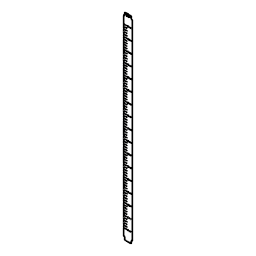
AG10 (Autodesk Fusion 360 design; units mm, degrees)
part number: 2025-10-06-13-20-48-967
Autodesk Fusion 360 part; units mm, degrees
(part 1 of 20)
sketch "Boceto1" plane through (0, 0, 0) normal (0, 1, 0) x (1, 0, 0)
  line L0 (0, 0) -> (40, 0)
  line L1 (40, 0) -> (40, 874)
  line L2 (40, 874) -> (0, 874)
  line L3 (0, 874) -> (0, 0)
  dimension "d1" = 40
  dimension "d2" = 874
  constraint horizontal L0
  constraint vertical L1
  constraint horizontal L2
  constraint vertical L3
  constraint coincident L0.start L3.end
  measures "d1" distance of L1.end L2.end
  measures "d2" distance of L0.end L1.end
extrude "Extruir1" add sketch "Boceto1" along normal blind 3
sketch "Boceto2" plane through (0, 0, 0) normal (0, -1, 0) x (1, 0, 0)
  line L0 (0, 0) -> (0, -874)
  line L1 (0, -874) -> (40, -874)
  line L2 (40, -874) -> (40, 0)
  line L3 (40, 0) -> (0, 0)
  line L4 (0, -836.5) -> (17.5, -836.5)
  line L5 (17.5, -836.5) -> (17.5, -837.5)
  line L6 (17.5, -837.5) -> (0, -837.5)
  line L7 (0, -836.5) -> (0, -837.5)
  line L8 (0, -836.5) -> (0, -837.5)
  line L9 (0, -826.5) -> (17.5, -826.5)
  line L10 (17.5, -827.5) -> (0, -827.5)
  line L11 (0, -826.5) -> (0, -827.5)
  line L12 (17.5, -826.5) -> (17.5, -827.5)
  line L13 (0, -816.5) -> (17.5, -816.5)
  line L14 (17.5, -817.5) -> (0, -817.5)
  line L15 (0, -816.5) -> (0, -817.5)
  line L16 (17.5, -816.5) -> (17.5, -817.5)
  line L17 (0, -806.5) -> (17.5, -806.5)
  line L18 (17.5, -807.5) -> (0, -807.5)
  line L19 (0, -806.5) -> (0, -807.5)
  line L20 (17.5, -806.5) -> (17.5, -807.5)
  line L21 (0, -796.5) -> (17.5, -796.5)
  line L22 (17.5, -797.5) -> (0, -797.5)
  line L23 (0, -796.5) -> (0, -797.5)
  line L24 (17.5, -796.5) -> (17.5, -797.5)
  line L25 (0, -786.5) -> (17.5, -786.5)
  line L26 (17.5, -787.5) -> (0, -787.5)
  line L27 (0, -786.5) -> (0, -787.5)
  line L28 (17.5, -786.5) -> (17.5, -787.5)
  line L29 (0, -776.5) -> (17.5, -776.5)
  line L30 (17.5, -777.5) -> (0, -777.5)
  line L31 (0, -776.5) -> (0, -777.5)
  line L32 (17.5, -776.5) -> (17.5, -777.5)
  line L33 (0, -766.5) -> (17.5, -766.5)
  line L34 (17.5, -767.5) -> (0, -767.5)
  line L35 (0, -766.5) -> (0, -767.5)
  line L36 (17.5, -766.5) -> (17.5, -767.5)
  line L37 (0, -756.5) -> (17.5, -756.5)
  line L38 (17.5, -757.5) -> (0, -757.5)
  line L39 (0, -756.5) -> (0, -757.5)
  line L40 (17.5, -756.5) -> (17.5, -757.5)
  line L41 (0, -746.5) -> (17.5, -746.5)
  line L42 (17.5, -747.5) -> (0, -747.5)
  line L43 (0, -746.5) -> (0, -747.5)
  line L44 (17.5, -746.5) -> (17.5, -747.5)
  line L45 (0, -736.5) -> (17.5, -736.5)
  line L46 (17.5, -737.5) -> (0, -737.5)
  line L47 (0, -736.5) -> (0, -737.5)
  line L48 (17.5, -736.5) -> (17.5, -737.5)
  line L49 (0, -726.5) -> (17.5, -726.5)
  line L50 (17.5, -727.5) -> (0, -727.5)
  line L51 (0, -726.5) -> (0, -727.5)
  line L52 (17.5, -726.5) -> (17.5, -727.5)
  line L53 (0, -716.5) -> (17.5, -716.5)
  line L54 (17.5, -717.5) -> (0, -717.5)
  line L55 (0, -716.5) -> (0, -717.5)
  line L56 (17.5, -716.5) -> (17.5, -717.5)
  line L57 (0, -706.5) -> (17.5, -706.5)
  line L58 (17.5, -707.5) -> (0, -707.5)
  line L59 (0, -706.5) -> (0, -707.5)
  line L60 (17.5, -706.5) -> (17.5, -707.5)
  line L61 (0, -696.5) -> (17.5, -696.5)
  line L62 (17.5, -697.5) -> (0, -697.5)
  line L63 (0, -696.5) -> (0, -697.5)
  line L64 (17.5, -696.5) -> (17.5, -697.5)
  line L65 (0, -686.5) -> (17.5, -686.5)
  line L66 (17.5, -687.5) -> (0, -687.5)
  line L67 (0, -686.5) -> (0, -687.5)
  line L68 (17.5, -686.5) -> (17.5, -687.5)
  line L69 (0, -676.5) -> (17.5, -676.5)
  line L70 (17.5, -677.5) -> (0, -677.5)
  line L71 (0, -676.5) -> (0, -677.5)
  line L72 (17.5, -676.5) -> (17.5, -677.5)
  line L73 (0, -666.5) -> (17.5, -666.5)
  line L74 (17.5, -667.5) -> (0, -667.5)
  line L75 (0, -666.5) -> (0, -667.5)
  line L76 (17.5, -666.5) -> (17.5, -667.5)
  line L77 (0, -656.5) -> (17.5, -656.5)
  line L78 (17.5, -657.5) -> (0, -657.5)
  line L79 (0, -656.5) -> (0, -657.5)
  line L80 (17.5, -656.5) -> (17.5, -657.5)
  line L81 (0, -646.5) -> (17.5, -646.5)
  line L82 (17.5, -647.5) -> (0, -647.5)
  line L83 (0, -646.5) -> (0, -647.5)
  line L84 (17.5, -646.5) -> (17.5, -647.5)
  line L85 (0, -636.5) -> (17.5, -636.5)
  line L86 (17.5, -637.5) -> (0, -637.5)
  line L87 (0, -636.5) -> (0, -637.5)
  line L88 (17.5, -636.5) -> (17.5, -637.5)
  line L89 (0, -626.5) -> (17.5, -626.5)
  line L90 (17.5, -627.5) -> (0, -627.5)
  line L91 (0, -626.5) -> (0, -627.5)
  line L92 (17.5, -626.5) -> (17.5, -627.5)
  line L93 (0, -616.5) -> (17.5, -616.5)
  line L94 (17.5, -617.5) -> (0, -617.5)
  line L95 (0, -616.5) -> (0, -617.5)
  line L96 (17.5, -616.5) -> (17.5, -617.5)
  line L97 (0, -606.5) -> (17.5, -606.5)
  line L98 (17.5, -607.5) -> (0, -607.5)
  line L99 (0, -606.5) -> (0, -607.5)
  line L100 (17.5, -606.5) -> (17.5, -607.5)
  line L101 (0, -596.5) -> (17.5, -596.5)
  line L102 (17.5, -597.5) -> (0, -597.5)
  line L103 (0, -596.5) -> (0, -597.5)
  line L104 (17.5, -596.5) -> (17.5, -597.5)
  line L105 (0, -586.5) -> (17.5, -586.5)
  line L106 (17.5, -587.5) -> (0, -587.5)
  line L107 (0, -586.5) -> (0, -587.5)
  line L108 (17.5, -586.5) -> (17.5, -587.5)
  line L109 (0, -576.5) -> (17.5, -576.5)
  line L110 (17.5, -577.5) -> (0, -577.5)
  line L111 (0, -576.5) -> (0, -577.5)
  line L112 (17.5, -576.5) -> (17.5, -577.5)
  line L113 (0, -566.5) -> (17.5, -566.5)
  line L114 (17.5, -567.5) -> (0, -567.5)
  line L115 (0, -566.5) -> (0, -567.5)
  line L116 (17.5, -566.5) -> (17.5, -567.5)
  line L117 (0, -556.5) -> (17.5, -556.5)
  line L118 (17.5, -557.5) -> (0, -557.5)
  line L119 (0, -556.5) -> (0, -557.5)
  line L120 (17.5, -556.5) -> (17.5, -557.5)
  line L121 (0, -546.5) -> (17.5, -546.5)
  line L122 (17.5, -547.5) -> (0, -547.5)
  line L123 (0, -546.5) -> (0, -547.5)
  line L124 (17.5, -546.5) -> (17.5, -547.5)
  line L125 (0, -536.5) -> (17.5, -536.5)
  line L126 (17.5, -537.5) -> (0, -537.5)
  line L127 (0, -536.5) -> (0, -537.5)
  line L128 (17.5, -536.5) -> (17.5, -537.5)
  line L129 (0, -526.5) -> (17.5, -526.5)
  line L130 (17.5, -527.5) -> (0, -527.5)
  line L131 (0, -526.5) -> (0, -527.5)
  line L132 (17.5, -526.5) -> (17.5, -527.5)
  line L133 (0, -516.5) -> (17.5, -516.5)
  line L134 (17.5, -517.5) -> (0, -517.5)
  line L135 (0, -516.5) -> (0, -517.5)
  line L136 (17.5, -516.5) -> (17.5, -517.5)
  line L137 (0, -506.5) -> (17.5, -506.5)
  line L138 (17.5, -507.5) -> (0, -507.5)
  line L139 (0, -506.5) -> (0, -507.5)
  line L140 (17.5, -506.5) -> (17.5, -507.5)
  line L141 (0, -496.5) -> (17.5, -496.5)
  line L142 (17.5, -497.5) -> (0, -497.5)
  line L143 (0, -496.5) -> (0, -497.5)
  line L144 (17.5, -496.5) -> (17.5, -497.5)
  line L145 (0, -486.5) -> (17.5, -486.5)
  line L146 (17.5, -487.5) -> (0, -487.5)
  line L147 (0, -486.5) -> (0, -487.5)
  line L148 (17.5, -486.5) -> (17.5, -487.5)
  line L149 (0, -476.5) -> (17.5, -476.5)
  line L150 (17.5, -477.5) -> (0, -477.5)
  line L151 (0, -476.5) -> (0, -477.5)
  line L152 (17.5, -476.5) -> (17.5, -477.5)
  line L153 (0, -466.5) -> (17.5, -466.5)
  line L154 (17.5, -467.5) -> (0, -467.5)
  line L155 (0, -466.5) -> (0, -467.5)
  line L156 (17.5, -466.5) -> (17.5, -467.5)
  line L157 (0, -456.5) -> (17.5, -456.5)
  line L158 (17.5, -457.5) -> (0, -457.5)
  line L159 (0, -456.5) -> (0, -457.5)
  line L160 (17.5, -456.5) -> (17.5, -457.5)
  line L161 (0, -446.5) -> (17.5, -446.5)
  line L162 (17.5, -447.5) -> (0, -447.5)
  line L163 (0, -446.5) -> (0, -447.5)
  line L164 (17.5, -446.5) -> (17.5, -447.5)
  line L165 (0, -436.5) -> (17.5, -436.5)
  line L166 (17.5, -437.5) -> (0, -437.5)
  line L167 (0, -436.5) -> (0, -437.5)
  line L168 (17.5, -436.5) -> (17.5, -437.5)
  line L169 (0, -426.5) -> (17.5, -426.5)
  line L170 (17.5, -427.5) -> (0, -427.5)
  line L171 (0, -426.5) -> (0, -427.5)
  line L172 (17.5, -426.5) -> (17.5, -427.5)
  line L173 (0, -416.5) -> (17.5, -416.5)
  line L174 (17.5, -417.5) -> (0, -417.5)
  line L175 (0, -416.5) -> (0, -417.5)
  line L176 (17.5, -416.5) -> (17.5, -417.5)
  line L177 (0, -406.5) -> (17.5, -406.5)
  line L178 (17.5, -407.5) -> (0, -407.5)
  line L179 (0, -406.5) -> (0, -407.5)
  line L180 (17.5, -406.5) -> (17.5, -407.5)
  line L181 (0, -396.5) -> (17.5, -396.5)
  line L182 (17.5, -397.5) -> (0, -397.5)
  line L183 (0, -396.5) -> (0, -397.5)
  line L184 (17.5, -396.5) -> (17.5, -397.5)
  line L185 (0, -386.5) -> (17.5, -386.5)
  line L186 (17.5, -387.5) -> (0, -387.5)
  line L187 (0, -386.5) -> (0, -387.5)
  line L188 (17.5, -386.5) -> (17.5, -387.5)
  line L189 (0, -376.5) -> (17.5, -376.5)
  line L190 (17.5, -377.5) -> (0, -377.5)
  line L191 (0, -376.5) -> (0, -377.5)
  line L192 (17.5, -376.5) -> (17.5, -377.5)
  line L193 (0, -366.5) -> (17.5, -366.5)
  line L194 (17.5, -367.5) -> (0, -367.5)
  line L195 (0, -366.5) -> (0, -367.5)
  line L196 (17.5, -366.5) -> (17.5, -367.5)
  line L197 (0, -356.5) -> (17.5, -356.5)
  line L198 (17.5, -357.5) -> (0, -357.5)
  line L199 (0, -356.5) -> (0, -357.5)
  line L200 (17.5, -356.5) -> (17.5, -357.5)
  line L201 (0, -346.5) -> (17.5, -346.5)
  line L202 (17.5, -347.5) -> (0, -347.5)
  line L203 (0, -346.5) -> (0, -347.5)
  line L204 (17.5, -346.5) -> (17.5, -347.5)
  line L205 (0, -336.5) -> (17.5, -336.5)
  line L206 (17.5, -337.5) -> (0, -337.5)
  line L207 (0, -336.5) -> (0, -337.5)
  line L208 (17.5, -336.5) -> (17.5, -337.5)
  line L209 (0, -326.5) -> (17.5, -326.5)
  line L210 (17.5, -327.5) -> (0, -327.5)
  line L211 (0, -326.5) -> (0, -327.5)
  line L212 (17.5, -326.5) -> (17.5, -327.5)
  line L213 (0, -316.5) -> (17.5, -316.5)
  line L214 (17.5, -317.5) -> (0, -317.5)
  line L215 (0, -316.5) -> (0, -317.5)
  line L216 (17.5, -316.5) -> (17.5, -317.5)
  line L217 (0, -306.5) -> (17.5, -306.5)
  line L218 (17.5, -307.5) -> (0, -307.5)
  line L219 (0, -306.5) -> (0, -307.5)
  line L220 (17.5, -306.5) -> (17.5, -307.5)
  line L221 (0, -296.5) -> (17.5, -296.5)
  line L222 (17.5, -297.5) -> (0, -297.5)
  line L223 (0, -296.5) -> (0, -297.5)
  line L224 (17.5, -296.5) -> (17.5, -297.5)
  line L225 (0, -286.5) -> (17.5, -286.5)
  line L226 (17.5, -287.5) -> (0, -287.5)
  line L227 (0, -286.5) -> (0, -287.5)
  line L228 (17.5, -286.5) -> (17.5, -287.5)
  line L229 (0, -276.5) -> (17.5, -276.5)
  line L230 (17.5, -277.5) -> (0, -277.5)
  line L231 (0, -276.5) -> (0, -277.5)
  line L232 (17.5, -276.5) -> (17.5, -277.5)
  line L233 (0, -266.5) -> (17.5, -266.5)
  line L234 (17.5, -267.5) -> (0, -267.5)
  line L235 (0, -266.5) -> (0, -267.5)
  line L236 (17.5, -266.5) -> (17.5, -267.5)
  line L237 (0, -256.5) -> (17.5, -256.5)
  line L238 (17.5, -257.5) -> (0, -257.5)
  line L239 (0, -256.5) -> (0, -257.5)
  line L240 (17.5, -256.5) -> (17.5, -257.5)
  line L241 (0, -246.5) -> (17.5, -246.5)
  line L242 (17.5, -247.5) -> (0, -247.5)
  line L243 (0, -246.5) -> (0, -247.5)
  line L244 (17.5, -246.5) -> (17.5, -247.5)
  line L245 (0, -236.5) -> (17.5, -236.5)
  line L246 (17.5, -237.5) -> (0, -237.5)
  line L247 (0, -236.5) -> (0, -237.5)
  line L248 (17.5, -236.5) -> (17.5, -237.5)
  line L249 (0, -226.5) -> (17.5, -226.5)
  line L250 (17.5, -227.5) -> (0, -227.5)
  line L251 (0, -226.5) -> (0, -227.5)
  line L252 (17.5, -226.5) -> (17.5, -227.5)
  line L253 (0, -216.5) -> (17.5, -216.5)
  line L254 (17.5, -217.5) -> (0, -217.5)
  line L255 (0, -216.5) -> (0, -217.5)
  line L256 (17.5, -216.5) -> (17.5, -217.5)
  line L257 (0, -206.5) -> (17.5, -206.5)
  line L258 (17.5, -207.5) -> (0, -207.5)
  line L259 (0, -206.5) -> (0, -207.5)
  line L260 (17.5, -206.5) -> (17.5, -207.5)
  line L261 (0, -196.5) -> (17.5, -196.5)
  line L262 (17.5, -197.5) -> (0, -197.5)
  line L263 (0, -196.5) -> (0, -197.5)
  line L264 (17.5, -196.5) -> (17.5, -197.5)
  line L265 (0, -186.5) -> (17.5, -186.5)
  line L266 (17.5, -187.5) -> (0, -187.5)
  line L267 (0, -186.5) -> (0, -187.5)
  line L268 (17.5, -186.5) -> (17.5, -187.5)
  line L269 (0, -176.5) -> (17.5, -176.5)
  line L270 (17.5, -177.5) -> (0, -177.5)
  line L271 (0, -176.5) -> (0, -177.5)
  line L272 (17.5, -176.5) -> (17.5, -177.5)
  line L273 (0, -166.5) -> (17.5, -166.5)
  line L274 (17.5, -167.5) -> (0, -167.5)
  line L275 (0, -166.5) -> (0, -167.5)
  line L276 (17.5, -166.5) -> (17.5, -167.5)
  line L277 (0, -156.5) -> (17.5, -156.5)
  line L278 (17.5, -157.5) -> (0, -157.5)
  line L279 (0, -156.5) -> (0, -157.5)
  line L280 (17.5, -156.5) -> (17.5, -157.5)
  line L281 (0, -146.5) -> (17.5, -146.5)
  line L282 (17.5, -147.5) -> (0, -147.5)
  line L283 (0, -146.5) -> (0, -147.5)
  line L284 (17.5, -146.5) -> (17.5, -147.5)
  line L285 (0, -136.5) -> (17.5, -136.5)
  line L286 (17.5, -137.5) -> (0, -137.5)
  line L287 (0, -136.5) -> (0, -137.5)
  line L288 (17.5, -136.5) -> (17.5, -137.5)
  line L289 (0, -126.5) -> (17.5, -126.5)
  line L290 (17.5, -127.5) -> (0, -127.5)
  line L291 (0, -126.5) -> (0, -127.5)
  line L292 (17.5, -126.5) -> (17.5, -127.5)
  line L293 (0, -116.5) -> (17.5, -116.5)
  line L294 (17.5, -117.5) -> (0, -117.5)
  line L295 (0, -116.5) -> (0, -117.5)
  line L296 (17.5, -116.5) -> (17.5, -117.5)
  line L297 (0, -106.5) -> (17.5, -106.5)
  line L298 (17.5, -107.5) -> (0, -107.5)
  line L299 (0, -106.5) -> (0, -107.5)
  line L300 (17.5, -106.5) -> (17.5, -107.5)
  line L301 (0, -96.5) -> (17.5, -96.5)
  line L302 (17.5, -97.5) -> (0, -97.5)
  line L303 (0, -96.5) -> (0, -97.5)
  line L304 (17.5, -96.5) -> (17.5, -97.5)
  line L305 (0, -86.5) -> (17.5, -86.5)
  line L306 (17.5, -87.5) -> (0, -87.5)
  line L307 (0, -86.5) -> (0, -87.5)
  line L308 (17.5, -86.5) -> (17.5, -87.5)
  line L309 (0, -76.5) -> (17.5, -76.5)
  line L310 (17.5, -77.5) -> (0, -77.5)
  line L311 (0, -76.5) -> (0, -77.5)
  line L312 (17.5, -76.5) -> (17.5, -77.5)
  line L313 (0, -66.5) -> (17.5, -66.5)
  line L314 (17.5, -67.5) -> (0, -67.5)
  line L315 (0, -66.5) -> (0, -67.5)
  line L316 (17.5, -66.5) -> (17.5, -67.5)
  line L317 (0, -56.5) -> (17.5, -56.5)
  line L318 (17.5, -57.5) -> (0, -57.5)
  line L319 (0, -56.5) -> (0, -57.5)
  line L320 (17.5, -56.5) -> (17.5, -57.5)
  line L321 (0, -46.5) -> (17.5, -46.5)
  line L322 (17.5, -47.5) -> (0, -47.5)
  line L323 (0, -46.5) -> (0, -47.5)
  line L324 (17.5, -46.5) -> (17.5, -47.5)
  line L325 (0, -837) -> (35, -837) construction
  line L326 (0, -827) -> (35, -827) construction
  line L327 (0, -817) -> (35, -817) construction
  line L328 (0, -807) -> (35, -807) construction
  line L329 (0, -797) -> (35, -797) construction
  line L330 (0, -787) -> (35, -787) construction
  line L331 (0, -777) -> (35, -777) construction
  line L332 (0, -767) -> (35, -767) construction
  line L333 (0, -757) -> (35, -757) construction
  line L334 (0, -747) -> (35, -747) construction
  line L335 (0, -737) -> (35, -737) construction
  line L336 (0, -727) -> (35, -727) construction
  line L337 (0, -717) -> (35, -717) construction
  line L338 (0, -707) -> (35, -707) construction
  line L339 (0, -697) -> (35, -697) construction
  line L340 (0, -687) -> (35, -687) construction
  line L341 (0, -677) -> (35, -677) construction
  line L342 (0, -667) -> (35, -667) construction
  line L343 (0, -657) -> (35, -657) construction
  line L344 (0, -647) -> (35, -647) construction
  line L345 (0, -637) -> (35, -637) construction
  line L346 (0, -627) -> (35, -627) construction
  line L347 (0, -617) -> (35, -617) construction
  line L348 (0, -607) -> (35, -607) construction
  line L349 (0, -597) -> (35, -597) construction
  line L350 (0, -587) -> (35, -587) construction
  line L351 (0, -577) -> (35, -577) construction
  line L352 (0, -567) -> (35, -567) construction
  line L353 (0, -557) -> (35, -557) construction
  line L354 (0, -547) -> (35, -547) construction
  line L355 (0, -537) -> (35, -537) construction
  line L356 (0, -527) -> (35, -527) construction
  line L357 (0, -517) -> (35, -517) construction
  line L358 (0, -507) -> (35, -507) construction
  line L359 (0, -497) -> (35, -497) construction
  line L360 (0, -487) -> (35, -487) construction
  line L361 (0, -477) -> (35, -477) construction
  line L362 (0, -467) -> (35, -467) construction
  line L363 (0, -457) -> (35, -457) construction
  line L364 (0, -447) -> (35, -447) construction
  line L365 (0, -437) -> (35, -437) construction
  line L366 (0, -427) -> (35, -427) construction
  line L367 (0, -417) -> (35, -417) construction
  line L368 (0, -407) -> (35, -407) construction
  line L369 (0, -397) -> (35, -397) construction
  line L370 (0, -387) -> (35, -387) construction
  line L371 (0, -377) -> (35, -377) construction
  line L372 (0, -367) -> (35, -367) construction
  line L373 (0, -357) -> (35, -357) construction
  line L374 (0, -347) -> (35, -347) construction
  line L375 (0, -337) -> (35, -337) construction
  line L376 (0, -327) -> (35, -327) construction
  line L377 (0, -317) -> (35, -317) construction
  line L378 (0, -307) -> (35, -307) construction
  line L379 (0, -297) -> (35, -297) construction
  line L380 (0, -287) -> (35, -287) construction
  line L381 (0, -277) -> (35, -277) construction
  line L382 (0, -267) -> (35, -267) construction
  line L383 (0, -257) -> (35, -257) construction
  line L384 (0, -247) -> (35, -247) construction
  line L385 (0, -237) -> (35, -237) construction
  line L386 (0, -227) -> (35, -227) construction
  line L387 (0, -217) -> (35, -217) construction
  line L388 (0, -207) -> (35, -207) construction
  line L389 (0, -197) -> (35, -197) construction
  line L390 (0, -187) -> (35, -187) construction
  line L391 (0, -177) -> (35, -177) construction
  line L392 (0, -167) -> (35, -167) construction
  line L393 (0, -157) -> (35, -157) construction
  line L394 (0, -147) -> (35, -147) construction
  line L395 (0, -137) -> (35, -137) construction
  line L396 (0, -127) -> (35, -127) construction
  line L397 (0, -117) -> (35, -117) construction
  line L398 (0, -107) -> (35, -107) construction
  line L399 (0, -97) -> (35, -97) construction
  line L400 (0, -87) -> (35, -87) construction
  line L401 (0, -77) -> (35, -77) construction
  line L402 (0, -67) -> (35, -67) construction
  line L403 (0, -57) -> (35, -57) construction
  line L404 (0, -47) -> (35, -47) construction
  line L405 (0, -36.5) -> (17.5, -36.5)
  line L406 (17.5, -37.5) -> (0, -37.5)
  line L407 (0, -36.5) -> (0, -37.5)
  line L408 (17.5, -36.5) -> (17.5, -37.5)
  line L409 (0, -37) -> (35, -37) construction
  dimension "d11" = 0
  dimension "d12" = 800
  dimension "d34" = 0
  dimension "d35" = 800
  constraint midpoint L8 L325.start
sketch "Boceto5" plane through (0, 0, 0) normal (0, -1, 0) x (1, 0, 0)
  line L0 (17.5002, -789) -> (35.0197, -788.9987) construction
  line L1 (35.0197, -788.9987) -> (35.0194, -784.9987) construction
  line L2 (35.0194, -784.9987) -> (17.4998, -785) construction
  line L3 (17.4998, -785) -> (17.5002, -789) construction
  line L4 (17.5, -739) -> (35.0058, -738.9996) construction
  line L5 (35.0058, -738.9996) -> (35.0057, -734.9996) construction
  line L6 (35.0057, -734.9996) -> (17.5, -735) construction
  line L7 (17.5, -735) -> (17.5, -739) construction
  line L8 (17.5, -689) -> (35.0027, -688.9998) construction
  line L9 (35.0027, -688.9998) -> (35.0027, -684.9998) construction
  line L10 (35.0027, -684.9998) -> (17.5, -685) construction
  line L11 (17.5, -685) -> (17.5, -689) construction
  line L12 (17.5001, -639) -> (35.0059, -638.9995) construction
  line L13 (35.0059, -638.9995) -> (35.0057, -634.9995) construction
  line L14 (35.0057, -634.9995) -> (17.4999, -635) construction
  line L15 (17.4999, -635) -> (17.5001, -639) construction
  line L16 (17.5, -589) -> (35.001, -588.9999) construction
  line L17 (35.001, -588.9999) -> (35.0009, -584.9999) construction
  line L18 (35.0009, -584.9999) -> (17.5, -585) construction
  line L19 (17.5, -585) -> (17.5, -589) construction
  line L20 (17.5002, -539) -> (35.0154, -538.9985) construction
  line L21 (35.0154, -538.9985) -> (35.015, -534.9985) construction
  line L22 (35.015, -534.9985) -> (17.4998, -535) construction
  line L23 (17.4998, -535) -> (17.5002, -539) construction
  line L24 (17.5, -489) -> (35.0025, -488.9997) construction
  line L25 (35.0025, -488.9997) -> (35.0025, -484.9997) construction
  line L26 (35.0025, -484.9997) -> (17.5, -485) construction
  line L27 (17.5, -485) -> (17.5, -489) construction
  line L28 (17.5002, -439) -> (35.0113, -438.9986) construction
  line L29 (35.0113, -438.9986) -> (35.0109, -434.9986) construction
  line L30 (35.0109, -434.9986) -> (17.4998, -435) construction
  line L31 (17.4998, -435) -> (17.5002, -439) construction
  line L32 (17.5, -389) -> (35.002, -388.9997) construction
  line L33 (35.002, -388.9997) -> (35.0019, -384.9997) construction
  line L34 (35.0019, -384.9997) -> (17.5, -385) construction
  line L35 (17.5, -385) -> (17.5, -389) construction
  line L36 (17.5001, -339) -> (35.0028, -338.9996) construction
  line L37 (35.0028, -338.9996) -> (35.0027, -334.9996) construction
  line L38 (35.0027, -334.9996) -> (17.4999, -335) construction
  line L39 (17.4999, -335) -> (17.5001, -339) construction
  line L40 (17.5, -289) -> (35.0002, -289) construction
  line L41 (35.0002, -289) -> (35.0002, -285) construction
  line L42 (35.0002, -285) -> (17.5, -285) construction
  line L43 (17.5, -285) -> (17.5, -289) construction
  line L44 (17.5, -239) -> (34.9994, -239.0001) construction
  line L45 (34.9994, -239.0001) -> (34.9994, -235.0001) construction
  line L46 (34.9994, -235.0001) -> (17.5, -235) construction
  line L47 (17.5, -235) -> (17.5, -239) construction
  line L48 (17.5, -189) -> (35, -189) construction
  line L49 (35, -189) -> (35, -185) construction
  line L50 (35, -185) -> (17.5, -185) construction
  line L51 (17.5, -185) -> (17.5, -189) construction
  line L52 (17.5, -139) -> (35, -139) construction
  line L53 (35, -139) -> (35, -135) construction
  line L54 (35, -135) -> (17.5, -135) construction
  line L55 (17.5, -135) -> (17.5, -139) construction
  line L56 (17.5, -89) -> (35, -89) construction
  line L57 (35, -89) -> (35, -85) construction
  line L58 (35, -85) -> (17.5, -85) construction
  line L59 (17.5, -85) -> (17.5, -89) construction
  line L60 (17.5, -39) -> (35, -39) construction
  line L61 (35, -39) -> (35, -35) construction
  line L62 (35, -35) -> (17.5, -35) construction
  line L63 (17.5, -35) -> (17.5, -39) construction
  line L64 (0, -827) -> (35, -827) construction
  line L65 (17.5001, -839) -> (35.0094, -838.9994) construction
  line L66 (35.0094, -838.9994) -> (35.0093, -834.9994) construction
  line L67 (35.0093, -834.9994) -> (17.4999, -835) construction
  line L68 (17.4999, -835) -> (17.5001, -839) construction
  dimension "d93" = 5
  dimension "d94" = 0
  dimension "d103" = 5
  dimension "d104" = 0
  dimension "d113" = 5
  dimension "d114" = 0
  dimension "d123" = 5
  dimension "d124" = 0
  dimension "d133" = 5
  dimension "d134" = 0
  dimension "d143" = 5
  dimension "d144" = 0
  dimension "d153" = 5
  dimension "d154" = 0
  dimension "d163" = 5
  dimension "d164" = 0
  dimension "d173" = 5
  dimension "d174" = 0
  dimension "d183" = 5
  dimension "d184" = 0
  dimension "d193" = 5
  dimension "d194" = 0
  dimension "d203" = 5
  dimension "d204" = 0
  dimension "d213" = 5
  dimension "d214" = 0
  dimension "d223" = 5
  dimension "d224" = 0
  dimension "d233" = 5
  dimension "d234" = 0
  dimension "d243" = 5
  dimension "d244" = 0
  dimension "d245" = 5
  dimension "d246" = 0
  text T0 "5 cm" font "Arial" height 5 align centre middle in box 17.5196 x 4 at (17.5002, -789) x (1, 0.000075) y (-0.000075, 1) spacing 1 kerned
  text T1 "10cm" font "Arial" height 5 align centre middle in box 17.5057 x 4 at (17.5, -739) x (1, 0.000024) y (-0.000024, 1) spacing 1 kerned
  text T2 "15cm" font "Arial" height 5 align centre middle in box 17.5027 x 4 at (17.5, -689) x (1, 0.000012) y (-0.000012, 1) spacing 1 kerned
  text T3 "20cm" font "Arial" height 5 align centre middle in box 17.5058 x 4 at (17.5001, -639) x (1, 0.000028) y (-0.000028, 1) spacing 1 kerned
  text T4 "25cm" font "Arial" height 5 align centre middle in box 17.501 x 4 at (17.5, -589) x (1, 0.000005) y (-0.000005, 1) spacing 1 kerned
  text T5 "30cm" font "Arial" height 5 align centre middle in box 17.5152 x 4 at (17.5002, -539) x (1, 0.000086) y (-0.000086, 1) spacing 1 kerned
  text T6 "35cm" font "Arial" height 5 align centre middle in box 17.5025 x 4 at (17.5, -489) x (1, 0.000016) y (-0.000016, 1) spacing 1 kerned
  text T7 "40cm" font "Arial" height 5 align centre middle in box 17.5111 x 4 at (17.5002, -439) x (1, 0.000077) y (-0.000077, 1) spacing 1 kerned
  text T8 "45cm" font "Arial" height 5 align centre middle in box 17.5019 x 4 at (17.5, -389) x (1, 0.000015) y (-0.000015, 1) spacing 1 kerned
  text T9 "50cm" font "Arial" height 5 align centre middle in box 17.5028 x 4 at (17.5001, -339) x (1, 0.000025) y (-0.000025, 1) spacing 1 kerned
  text T10 "55cm" font "Arial" height 5 align centre middle in box 17.5002 x 4 at (17.5, -289) x (1, 0.000002) y (-0.000002, 1) spacing 1 kerned
  text T11 "60cm" font "Arial" height 5 align centre middle in box 17.4994 x 4 at (17.5, -239) x (1, -0.000008) y (0.000008, 1) spacing 1 kerned
  text T12 "65cm" font "Arial" height 5 align centre middle in box 17.5 x 4 at (17.5, -189) x (1, 0) y (0, 1) spacing 1 kerned
  text T13 "70cm" font "Arial" height 5 align centre middle in box 17.5 x 4 at (17.5, -139) x (1, -0.000001) y (0.000001, 1) spacing 1 kerned
  text T14 "75cm" font "Arial" height 5 align centre middle in box 17.5 x 4 at (17.5, -89) x (1, 0.000001) y (-0.000001, 1) spacing 1 kerned
  text T15 "80cm" font "Arial" height 5 align centre middle in box 17.5 x 4 at (17.5, -39) x (1, -0.000001) y (0.000001, 1) spacing 1 kerned
  text T16 "0 cm" font "Arial" height 5 align centre middle in box 17.5094 x 4 at (17.5001, -839) x (1, 0.000035) y (-0.000035, 1) spacing 1 kerned
sketch "Boceto6" plane through (0, 0, 0) normal (0, -1, 0) x (1, 0, 0)
  line L0 (0, 0) -> (0, -874)
  line L1 (0, -874) -> (40, -874)
  line L2 (40, -874) -> (40, 0)
  line L3 (40, 0) -> (0, 0)
  line L4 (40, 0) -> (35, 0)
  line L5 (35, 0) -> (35, -3)
  line L6 (35, -3) -> (40, -3)
  line L7 (40, -3) -> (40, 0)
  line L8 (0, 0) -> (5, 0)
  line L9 (5, 0) -> (5, -3)
  line L10 (5, -3) -> (0, -3)
  line L11 (0, -3) -> (0, 0)
  constraint horizontal L4
  constraint vertical L5
  constraint horizontal L6
  constraint vertical L7
  constraint coincident L2.end L3.start
  constraint horizontal L8
  constraint vertical L9
  constraint horizontal L10
  constraint vertical L11
  constraint coincident L0.start L3.end
extrude "Extruir3" cut sketch "Boceto6" against normal blind 3 contours L0 L3 L8 L9 L10 L11 | L2 L3 L4 L5 L6 L7
sketch "Boceto7" plane through (0, 0, 0) normal (0, -1, 0) x (1, 0, 0)
  line L0 (5, -3) -> (0, -3)
  line L1 (0, -3) -> (0, -874)
  line L2 (0, -874) -> (40, -874)
  line L3 (40, -874) -> (40, -3)
  line L4 (40, -3) -> (35, -3)
  line L5 (35, -3) -> (35, 0)
  line L6 (35, 0) -> (5, 0)
  line L7 (5, 0) -> (5, -3)
  line L8 (40, -874) -> (35, -874)
  line L9 (35, -874) -> (35, -870.7)
  line L10 (35, -870.7) -> (40, -870.7)
  line L11 (40, -870.7) -> (40, -874)
  line L12 (0, -874) -> (5, -874)
  line L13 (5, -874) -> (5, -870.7)
  line L14 (5, -870.7) -> (0, -870.7)
  line L15 (0, -870.7) -> (0, -874)
  dimension "d251" = 5
  dimension "d252" = 5
  dimension "d255" = 3.3
  dimension "d256" = 3.3
  constraint horizontal L8
  constraint vertical L9
  constraint horizontal L10
  constraint vertical L11
  constraint coincident L2.end L3.start
  constraint horizontal L12
  constraint vertical L13
  constraint horizontal L14
  constraint vertical L15
  constraint coincident L1.end L2.start
  measures "d251" distance of L13.end L14.end
  measures "d252" distance of L9.end L10.end
  measures "d255" distance of L2.end L10.end
  measures "d256" distance of L1.end L14.end
extrude "Extruir4" cut sketch "Boceto7" along normal mid plane 40 contours L1 L2 L12 L13 L14 L15 | L2 L3 L8 L9 L10 L11
sketch "Boceto8" plane through (0, 0, 0) normal (0, 1, 0) x (1, 0, 0)
extrude "Extruir5" add sketch "Boceto2" along normal blind 1 contours L0 L1 L2 L3 L4 L5 L6 L9 L10 L12 L13 L14 L16 L17 L18 L20 L21 L22 L24 L25 L26 L28 L29 L30 L32 L33 L34 L36 L37 L38 L40 L41 L42 L44 L45 L46 L48 L49 L50 L52 L53 L54 L56 L57 L58 L60 L61 L62 L64 L65 L66 L68 L69 L70 L72 L73 L74 L76 L77 L78 L80 L81 L82 L84 L85 L86 L88 L89 L90 L92 L93 L94 L96 L97 L98 L100 L101 L102 L104 L105 L106 L108 L109 L110 L112 L113 L114 L116 L117 L118 L120 L121 L122 L124 L125 L126 L128 L129 L130 L132 L133 L134 L136 L137 L138 L140 L141 L142 L144 L145 L146 L148 L149 L150 L152 L153 L154 L156 L157 L158 L160 L161 L162 L164 L165 L166 L168 L169 L170 L172 L173 L174 L176 L177 L178 L180 L181 L182 L184 L185 L186 L188 L189 L190 L192 L193 L194 L196 L197 L198 L200 L201 L202 L204 L205 L206 L208 L209 L210 L212 L213 L214 L216 L217 L218 L220 L221 L222 L224 L225 L226 L228 L229 L230 L232 L233 L234 L236 L237 L238 L240 L241 L242 L244 L245 L246 L248 L249 L250 L252 L253 L254 L256 L257 L258 L260 L261 L262 L264 L265 L266 L268 L269 L270 L272 L273 L274 L276 L277 L278 L280 L281 L282 L284 L285 L286 L288 L289 L290 L292 L293 L294 L296 L297 L298 L300 L301 L302 L304 L305 L306 L308 L309 L310 L312 L313 L314 L316 L317 L318 L320 L321 L322 L324 L405 L406 L408
extrude "Extruir6" cut 1 faces at (25, 3, -292.2333) along direction (0, -1, 0) blind 1
extrude "Extruir7" cut sketch "Boceto5" along normal blind 1 text T15 T14 T13 T12 T11 T10 T9 T8 T7 T6 T5 T4 T3 T2 T1 T0 T16
extrude "Extruir8" cut 4 faces at (3.3333, 0, -871.8) (36.6667, 0, -871.8) (1.6667, 0, -1) (36.6667, 0, -1) along direction (0, -1, 0) blind 20
sketch "Boceto10" plane through (0, -1, 0) normal (0, -1, 0) x (1, 0, 0)
  line L0 (28.545, -839.4996) -> (28.5449, -835.8775)
  line L1 (28.5449, -835.8775) -> (29.094, -835.8775)
  line L2 (29.094, -835.8775) -> (29.094, -836.3857)
  spline S0 degree 3 poles (29.094, -836.3857) (29.1559, -836.3011) (29.2808, -836.1306) (29.4582, -836.0156) (29.5476, -835.9576) knots 0 0 0 0 0.031158 0.062835 0.062835 0.062835 0.062835
  spline S1 degree 3 poles (29.5476, -835.9576) (29.6468, -835.9104) (29.8507, -835.8133) (30.0763, -835.8016) (30.1922, -835.7956) knots 0 0 0 0 0.032617 0.067048 0.067048 0.067048 0.067048
  spline S2 degree 3 poles (30.1922, -835.7956) (30.3167, -835.8003) (30.5491, -835.8092) (30.7561, -835.914) (30.8522, -835.9627) knots 0 0 0 0 0.036859 0.068796 0.068796 0.068796 0.068796
  spline S3 degree 3 poles (30.8522, -835.9627) (30.9319, -836.0244) (31.0928, -836.1491) (31.1743, -836.3357) (31.2154, -836.4299) knots 0 0 0 0 0.029725 0.060035 0.060035 0.060035 0.060035
  spline S4 degree 3 poles (31.2154, -836.4299) (31.3656, -836.245) (31.6567, -835.8864) (32.1131, -835.8252) (32.3341, -835.7955) knots 0 0 0 0 0.068625 0.133024 0.133024 0.133024 0.133024
  spline S5 degree 3 poles (32.3341, -835.7955) (32.4992, -835.8039) (32.8071, -835.8196) (33.0502, -836.007) (33.1629, -836.0939) knots 0 0 0 0 0.048244 0.08997 0.08997 0.08997 0.08997
  spline S6 degree 3 poles (33.1629, -836.0939) (33.2472, -836.2162) (33.4366, -836.4911) (33.4471, -836.8268) (33.4528, -837.0131) knots 0 0 0 0 0.043695 0.098195 0.098195 0.098195 0.098195
  line L3 (33.4528, -837.0131) -> (33.4529, -839.4994)
  line L4 (33.4529, -839.4994) -> (32.8424, -839.4995)
  line L5 (32.8424, -839.4995) -> (32.8423, -837.2177)
  spline S7 degree 3 poles (32.8423, -837.2177) (32.8423, -837.1115) (32.8423, -836.9322) (32.7999, -836.7583) (32.7826, -836.6874) knots 0 0 0 0 0.031711 0.053535 0.053535 0.053535 0.053535
  spline S8 degree 3 poles (32.7826, -836.6874) (32.7582, -836.6357) (32.7084, -836.5303) (32.6141, -836.4615) (32.5661, -836.4265) knots 0 0 0 0 0.016863 0.034394 0.034394 0.034394 0.034394
  spline S9 degree 3 poles (32.5661, -836.4265) (32.5103, -836.3976) (32.3949, -836.3379) (32.2649, -836.3311) (32.1977, -836.3276) knots 0 0 0 0 0.018597 0.038532 0.038532 0.038532 0.038532
  spline S10 degree 3 poles (32.1977, -836.3276) (32.0766, -836.3374) (31.8386, -836.3566) (31.654, -836.5076) (31.5633, -836.5817) knots 0 0 0 0 0.035532 0.069798 0.069798 0.069798 0.069798
  spline S11 degree 3 poles (31.5633, -836.5817) (31.49, -836.6884) (31.3229, -836.9316) (31.3153, -837.2285) (31.311, -837.3951) knots 0 0 0 0 0.038079 0.086792 0.086792 0.086792 0.086792
  line L6 (31.311, -837.3951) -> (31.311, -839.4995)
  line L7 (31.311, -839.4995) -> (30.6971, -839.4995)
  line L8 (30.6971, -839.4995) -> (30.697, -837.1462)
  spline S12 degree 3 poles (30.697, -837.1462) (30.6946, -837.0241) (30.6903, -836.8074) (30.5906, -836.6159) (30.547, -836.5323) knots 0 0 0 0 0.036008 0.063954 0.063954 0.063954 0.063954
  spline S13 degree 3 poles (30.547, -836.5323) (30.4847, -836.4727) (30.3485, -836.3423) (30.1589, -836.3328) (30.0558, -836.3277) knots 0 0 0 0 0.025037 0.054812 0.054812 0.054812 0.054812
  spline S14 degree 3 poles (30.0558, -836.3277) (29.9711, -836.3333) (29.8016, -836.3447) (29.6516, -836.4243) (29.5766, -836.4641) knots 0 0 0 0 0.025172 0.050327 0.050327 0.050327 0.050327
  spline S15 degree 3 poles (29.5766, -836.4641) (29.508, -836.5158) (29.3677, -836.6214) (29.2949, -836.7814) (29.2577, -836.8631) knots 0 0 0 0 0.025339 0.051812 0.051812 0.051812 0.051812
  spline S16 degree 3 poles (29.2577, -836.8631) (29.229, -836.9694) (29.1622, -837.217) (29.1601, -837.4738) (29.1589, -837.6203) knots 0 0 0 0 0.032907 0.076633 0.076633 0.076633 0.076633
  line L9 (29.1589, -837.6203) -> (29.1589, -839.4996)
  line L10 (29.1589, -839.4996) -> (28.545, -839.4996)
  line L11 (19.0617, -788.1561) -> (19.7063, -788.1015)
  spline S17 degree 3 poles (19.7063, -788.1015) (19.734, -788.2447) (19.7853, -788.5096) (19.9591, -788.7149) (20.0389, -788.8091) knots 0 0 0 0 0.042908 0.079365 0.079365 0.079365 0.079365
  spline S18 degree 3 poles (20.0389, -788.8091) (20.1311, -788.8783) (20.3177, -789.0182) (20.5504, -789.0368) (20.6682, -789.0461) knots 0 0 0 0 0.033826 0.068485 0.068485 0.068485 0.068485
  spline S19 degree 3 poles (20.6682, -789.0461) (20.8106, -789.0318) (21.0974, -789.003) (21.311, -788.8093) (21.4185, -788.7118) knots 0 0 0 0 0.041772 0.0841 0.0841 0.0841 0.0841
  spline S20 degree 3 poles (21.4185, -788.7118) (21.508, -788.5868) (21.6971, -788.3223) (21.7156, -787.9967) (21.7254, -787.825) knots 0 0 0 0 0.045186 0.095569 0.095569 0.095569 0.095569
  spline S21 degree 3 poles (21.7254, -787.825) (21.7163, -787.6627) (21.6992, -787.3564) (21.5163, -787.1114) (21.4303, -786.9963) knots 0 0 0 0 0.047557 0.089725 0.089725 0.089725 0.089725
  spline S22 degree 3 poles (21.4303, -786.9963) (21.3218, -786.9078) (21.0972, -786.7246) (20.8075, -786.7036) (20.6578, -786.6928) knots 0 0 0 0 0.040971 0.08482 0.08482 0.08482 0.08482
  spline S23 degree 3 poles (20.6578, -786.6928) (20.5622, -786.6979) (20.3748, -786.708) (20.2053, -786.7883) (20.1223, -786.8275) knots 0 0 0 0 0.028423 0.055689 0.055689 0.055689 0.055689
  spline S24 degree 3 poles (20.1223, -786.8275) (20.0475, -786.8751) (19.9006, -786.9683) (19.7977, -787.1085) (19.7472, -787.1772) knots 0 0 0 0 0.026342 0.051681 0.051681 0.051681 0.051681
  line L12 (19.7472, -787.1772) -> (19.1708, -787.1022)
  line L13 (19.1708, -787.1022) -> (19.6549, -784.5339)
  line L14 (19.6549, -784.5339) -> (22.1413, -784.5337)
  line L15 (22.1413, -784.5337) -> (22.1413, -785.1204)
  line L16 (22.1413, -785.1204) -> (20.1461, -785.1205)
  line L17 (20.1461, -785.1205) -> (19.8767, -786.4643)
  spline S25 degree 3 poles (19.8767, -786.4643) (20.0262, -786.3728) (20.3171, -786.1948) (20.6565, -786.165) (20.8215, -786.1505) knots 0 0 0 0 0.051785 0.100763 0.100763 0.100763 0.100763
  spline S26 degree 3 poles (20.8215, -786.1505) (21.0307, -786.1688) (21.4463, -786.2053) (21.7672, -786.4717) (21.9265, -786.604) knots 0 0 0 0 0.061424 0.122014 0.122014 0.122014 0.122014
  spline S27 degree 3 poles (21.9265, -786.604) (22.0578, -786.7694) (22.3287, -787.1108) (22.3605, -787.5461) (22.3768, -787.7704) knots 0 0 0 0 0.061868 0.127641 0.127641 0.127641 0.127641
  spline S28 degree 3 poles (22.3768, -787.7704) (22.3616, -787.9874) (22.3318, -788.4132) (22.0967, -788.7691) (21.9813, -788.9437) knots 0 0 0 0 0.064036 0.125703 0.125703 0.125703 0.125703
  spline S29 degree 3 poles (21.9813, -788.9437) (21.8036, -789.1208) (21.4405, -789.4825) (20.9292, -789.5278) (20.6682, -789.5509) knots 0 0 0 0 0.072854 0.148822 0.148822 0.148822 0.148822
  spline S30 degree 3 poles (20.6682, -789.5509) (20.455, -789.5382) (20.0475, -789.5138) (19.7138, -789.2803) (19.5546, -789.169) knots 0 0 0 0 0.062678 0.119794 0.119794 0.119794 0.119794
  spline S31 degree 3 poles (19.5546, -789.169) (19.426, -789.0286) (19.1617, -788.7403) (19.0956, -788.3542) (19.0617, -788.1561) knots 0 0 0 0 0.055877 0.114795 0.114795 0.114795 0.114795
  line L18 (27.4212, -788.1384) -> (28.0249, -788.2168)
  spline S32 degree 3 poles (28.0249, -788.2168) (27.9822, -788.4107) (27.9005, -788.7824) (27.6421, -789.0608) (27.5185, -789.194) knots 0 0 0 0 0.058356 0.111856 0.111856 0.111856 0.111856
  spline S33 degree 3 poles (27.5185, -789.194) (27.3724, -789.2969) (27.0723, -789.5084) (26.7057, -789.5339) (26.5175, -789.5471) knots 0 0 0 0 0.052559 0.107965 0.107965 0.107965 0.107965
  spline S34 degree 3 poles (26.5175, -789.5471) (26.2844, -789.5296) (25.8328, -789.4957) (25.4886, -789.2028) (25.322, -789.0611) knots 0 0 0 0 0.068154 0.132052 0.132052 0.132052 0.132052
  spline S35 degree 3 poles (25.322, -789.0611) (25.1905, -788.8704) (24.9026, -788.453) (24.8815, -787.9442) (24.87, -787.6679) knots 0 0 0 0 0.068157 0.149141 0.149141 0.149141 0.149141
  spline S36 degree 3 poles (24.87, -787.6679) (24.8763, -787.4827) (24.8883, -787.1302) (25.0077, -786.7986) (25.0643, -786.6413) knots 0 0 0 0 0.055211 0.105055 0.105055 0.105055 0.105055
  spline S37 degree 3 poles (25.0643, -786.6413) (25.1365, -786.5044) (25.2787, -786.2348) (25.5316, -786.0649) (25.656, -785.9813) knots 0 0 0 0 0.04564 0.089884 0.089884 0.089884 0.089884
  spline S38 degree 3 poles (25.656, -785.9813) (25.792, -785.9171) (26.0658, -785.7878) (26.3683, -785.7701) (26.5206, -785.7612) knots 0 0 0 0 0.044643 0.089955 0.089955 0.089955 0.089955
  spline S39 degree 3 poles (26.5206, -785.7612) (26.7043, -785.7706) (27.0522, -785.7884) (27.3468, -785.9726) (27.4858, -786.0596) knots 0 0 0 0 0.054149 0.102527 0.102527 0.102527 0.102527
  spline S40 degree 3 poles (27.4858, -786.0596) (27.6003, -786.1731) (27.8394, -786.4101) (27.9232, -786.7368) (27.9668, -786.9071) knots 0 0 0 0 0.047449 0.099081 0.099081 0.099081 0.099081
  line L19 (27.9668, -786.9071) -> (27.3699, -786.9992)
  spline S41 degree 3 poles (27.3699, -786.9992) (27.3391, -786.8878) (27.2816, -786.6804) (27.1356, -786.523) (27.0681, -786.4501) knots 0 0 0 0 0.034086 0.063475 0.063475 0.063475 0.063475
  spline S42 degree 3 poles (27.0681, -786.4501) (26.9911, -786.3964) (26.8338, -786.2867) (26.6423, -786.273) (26.5445, -786.266) knots 0 0 0 0 0.027619 0.056426 0.056426 0.056426 0.056426
  spline S43 degree 3 poles (26.5445, -786.266) (26.3979, -786.2791) (26.1087, -786.3048) (25.8958, -786.5016) (25.7908, -786.5986) knots 0 0 0 0 0.04285 0.084486 0.084486 0.084486 0.084486
  spline S44 degree 3 poles (25.7908, -786.5986) (25.7066, -786.7382) (25.5128, -787.0597) (25.5052, -787.4372) (25.501, -787.6508) knots 0 0 0 0 0.048123 0.11083 0.11083 0.11083 0.11083
  spline S45 degree 3 poles (25.501, -787.6508) (25.5046, -787.8666) (25.5109, -788.2453) (25.6995, -788.5712) (25.7807, -788.7115) knots 0 0 0 0 0.063398 0.111295 0.111295 0.111295 0.111295
  spline S46 degree 3 poles (25.7807, -788.7115) (25.8819, -788.808) (26.0864, -789.0031) (26.3682, -789.0291) (26.5106, -789.0423) knots 0 0 0 0 0.040675 0.082263 0.082263 0.082263 0.082263
  spline S47 degree 3 poles (26.5106, -789.0423) (26.625, -789.0341) (26.8478, -789.018) (27.0271, -788.8852) (27.1143, -788.8205) knots 0 0 0 0 0.033628 0.065508 0.065508 0.065508 0.065508
  spline S48 degree 3 poles (27.1143, -788.8205) (27.1883, -788.7306) (27.3518, -788.5319) (27.3967, -788.2775) (27.4212, -788.1384) knots 0 0 0 0 0.034396 0.07593 0.07593 0.07593 0.07593
  spline S49 degree 3 poles (21.7321, -737.034) (21.7357, -736.7657) (21.7422, -736.2825) (21.8615, -735.8147) (21.9145, -735.6066) knots 0 0 0 0 0.080152 0.144341 0.144341 0.144341 0.144341
  spline S50 degree 3 poles (21.9145, -735.6066) (21.9791, -735.4398) (22.1017, -735.1233) (22.3428, -734.8853) (22.4568, -734.7727) knots 0 0 0 0 0.052977 0.10048 0.10048 0.10048 0.10048
  spline S51 degree 3 poles (22.4568, -734.7727) (22.5882, -734.6872) (22.863, -734.5083) (23.1911, -734.4893) (23.3623, -734.4794) knots 0 0 0 0 0.046203 0.096661 0.096661 0.096661 0.096661
  spline S52 degree 3 poles (23.3623, -734.4794) (23.4901, -734.485) (23.7356, -734.4957) (23.9605, -734.5941) (24.0683, -734.6414) knots 0 0 0 0 0.037989 0.072993 0.072993 0.072993 0.072993
  spline S53 degree 3 poles (24.0683, -734.6414) (24.1655, -734.7021) (24.3629, -734.8252) (24.5001, -735.0132) (24.5697, -735.1086) knots 0 0 0 0 0.034048 0.069103 0.069103 0.069103 0.069103
  spline S54 degree 3 poles (24.5697, -735.1086) (24.633, -735.2196) (24.767, -735.4545) (24.841, -735.7148) (24.8801, -735.8521) knots 0 0 0 0 0.038176 0.080832 0.080832 0.080832 0.080832
  spline S55 degree 3 poles (24.8801, -735.8521) (24.9128, -736.0232) (24.9874, -736.4133) (24.9907, -736.8107) (24.9926, -737.0339) knots 0 0 0 0 0.052146 0.118926 0.118926 0.118926 0.118926
  spline S56 degree 3 poles (24.9926, -737.0339) (24.989, -737.3005) (24.9824, -737.7813) (24.8645, -738.247) (24.8119, -738.4544) knots 0 0 0 0 0.079639 0.143634 0.143634 0.143634 0.143634
  spline S57 degree 3 poles (24.8119, -738.4544) (24.7477, -738.6214) (24.6259, -738.9384) (24.3852, -739.1771) (24.2713, -739.2901) knots 0 0 0 0 0.052961 0.100531 0.100531 0.100531 0.100531
  spline S58 degree 3 poles (24.2713, -739.2901) (24.1397, -739.3761) (23.864, -739.5562) (23.5346, -739.5752) (23.3624, -739.5851) knots 0 0 0 0 0.046339 0.097057 0.097057 0.097057 0.097057
  spline S59 degree 3 poles (23.3624, -739.5851) (23.1362, -739.5658) (22.6949, -739.5281) (22.3801, -739.2179) (22.2267, -739.0667) knots 0 0 0 0 0.065835 0.128409 0.128409 0.128409 0.128409
  spline S60 degree 3 poles (22.2267, -739.0667) (22.0832, -738.7986) (21.7456, -738.1676) (21.737, -737.4479) (21.7321, -737.034) knots 0 0 0 0 0.090022 0.211899 0.211899 0.211899 0.211899
  line L20 (28.1509, -738.173) -> (28.7546, -738.2514)
  spline S61 degree 3 poles (28.7546, -738.2514) (28.7119, -738.4453) (28.6302, -738.8171) (28.3717, -739.0954) (28.2481, -739.2286) knots 0 0 0 0 0.058356 0.111856 0.111856 0.111856 0.111856
  spline S62 degree 3 poles (28.2481, -739.2286) (28.1021, -739.3315) (27.802, -739.543) (27.4353, -739.5685) (27.2471, -739.5816) knots 0 0 0 0 0.052559 0.107965 0.107965 0.107965 0.107965
  spline S63 degree 3 poles (27.2471, -739.5816) (27.0141, -739.5641) (26.5625, -739.5302) (26.2182, -739.2373) (26.0517, -739.0956) knots 0 0 0 0 0.068154 0.132052 0.132052 0.132052 0.132052
  spline S64 degree 3 poles (26.0517, -739.0956) (25.9201, -738.9049) (25.6323, -738.4875) (25.6112, -737.9787) (25.5997, -737.7024) knots 0 0 0 0 0.068157 0.149141 0.149141 0.149141 0.149141
  spline S65 degree 3 poles (25.5997, -737.7024) (25.6061, -737.5171) (25.6181, -737.1646) (25.7375, -736.8331) (25.7941, -736.6758) knots 0 0 0 0 0.055211 0.105055 0.105055 0.105055 0.105055
  spline S66 degree 3 poles (25.7941, -736.6758) (25.8663, -736.5389) (26.0085, -736.2693) (26.2614, -736.0994) (26.3859, -736.0158) knots 0 0 0 0 0.04564 0.089884 0.089884 0.089884 0.089884
  spline S67 degree 3 poles (26.3859, -736.0158) (26.5218, -735.9516) (26.7957, -735.8223) (27.0981, -735.8047) (27.2505, -735.7958) knots 0 0 0 0 0.044643 0.089956 0.089956 0.089956 0.089956
  spline S68 degree 3 poles (27.2505, -735.7958) (27.4342, -735.8052) (27.7821, -735.8229) (28.0767, -736.0072) (28.2157, -736.0942) knots 0 0 0 0 0.054149 0.102527 0.102527 0.102527 0.102527
  spline S69 degree 3 poles (28.2157, -736.0942) (28.3301, -736.2077) (28.5692, -736.4447) (28.6529, -736.7715) (28.6966, -736.9417) knots 0 0 0 0 0.047449 0.099081 0.099081 0.099081 0.099081
  line L21 (28.6966, -736.9417) -> (28.0997, -737.0338)
  spline S70 degree 3 poles (28.0997, -737.0338) (28.0689, -736.9224) (28.0114, -736.715) (27.8654, -736.5576) (27.7979, -736.4847) knots 0 0 0 0 0.034086 0.063475 0.063475 0.063475 0.063475
  spline S71 degree 3 poles (27.7979, -736.4847) (27.7209, -736.431) (27.5636, -736.3213) (27.3721, -736.3076) (27.2743, -736.3006) knots 0 0 0 0 0.027619 0.056426 0.056426 0.056426 0.056426
  spline S72 degree 3 poles (27.2743, -736.3006) (27.1277, -736.3136) (26.8385, -736.3393) (26.6256, -736.5361) (26.5206, -736.6331) knots 0 0 0 0 0.04285 0.084486 0.084486 0.084486 0.084486
  spline S73 degree 3 poles (26.5206, -736.6331) (26.4364, -736.7727) (26.2425, -737.0942) (26.235, -737.4717) (26.2307, -737.6853) knots 0 0 0 0 0.048123 0.11083 0.11083 0.11083 0.11083
  spline S74 degree 3 poles (26.2307, -737.6853) (26.2343, -737.9011) (26.2406, -738.2798) (26.4292, -738.6057) (26.5104, -738.746) knots 0 0 0 0 0.063398 0.111295 0.111295 0.111295 0.111295
  spline S75 degree 3 poles (26.5104, -738.746) (26.6116, -738.8425) (26.8161, -739.0376) (27.0979, -739.0637) (27.2403, -739.0768) knots 0 0 0 0 0.040675 0.082263 0.082263 0.082263 0.082263
  spline S76 degree 3 poles (27.2403, -739.0768) (27.3547, -739.0686) (27.5775, -739.0526) (27.7568, -738.9198) (27.844, -738.8551) knots 0 0 0 0 0.033628 0.065508 0.065508 0.065508 0.065508
  spline S77 degree 3 poles (27.844, -738.8551) (27.918, -738.7651) (28.0815, -738.5665) (28.1264, -738.3121) (28.1509, -738.173) knots 0 0 0 0 0.034396 0.07593 0.07593 0.07593 0.07593
  line L22 (21.7306, -688.1902) -> (22.3752, -688.1357)
  spline S78 degree 3 poles (22.3752, -688.1357) (22.4029, -688.2789) (22.4541, -688.5438) (22.6279, -688.7491) (22.7077, -688.8434) knots 0 0 0 0 0.042908 0.079365 0.079365 0.079365 0.079365
  spline S79 degree 3 poles (22.7077, -688.8434) (22.7999, -688.9125) (22.9865, -689.0525) (23.2192, -689.071) (23.337, -689.0804) knots 0 0 0 0 0.033826 0.068485 0.068485 0.068485 0.068485
  spline S80 degree 3 poles (23.337, -689.0804) (23.4794, -689.0661) (23.7662, -689.0373) (23.9798, -688.8436) (24.0873, -688.7462) knots 0 0 0 0 0.041772 0.0841 0.0841 0.0841 0.0841
  spline S81 degree 3 poles (24.0873, -688.7462) (24.1768, -688.6211) (24.366, -688.3566) (24.3845, -688.031) (24.3943, -687.8594) knots 0 0 0 0 0.045186 0.095569 0.095569 0.095569 0.095569
  spline S82 degree 3 poles (24.3943, -687.8594) (24.3852, -687.697) (24.3681, -687.3907) (24.1852, -687.1457) (24.0992, -687.0306) knots 0 0 0 0 0.047557 0.089725 0.089725 0.089725 0.089725
  spline S83 degree 3 poles (24.0992, -687.0306) (23.9907, -686.9421) (23.7662, -686.7589) (23.4765, -686.7379) (23.3267, -686.7271) knots 0 0 0 0 0.040971 0.08482 0.08482 0.08482 0.08482
  spline S84 degree 3 poles (23.3267, -686.7271) (23.2311, -686.7322) (23.0437, -686.7423) (22.8742, -686.8225) (22.7912, -686.8618) knots 0 0 0 0 0.028423 0.055689 0.055689 0.055689 0.055689
  spline S85 degree 3 poles (22.7912, -686.8618) (22.7164, -686.9093) (22.5695, -687.0026) (22.4666, -687.1427) (22.4161, -687.2114) knots 0 0 0 0 0.026342 0.051681 0.051681 0.051681 0.051681
  line L23 (22.4161, -687.2114) -> (21.8397, -687.1364)
  line L24 (21.8397, -687.1364) -> (22.324, -684.5681)
  line L25 (22.324, -684.5681) -> (24.8103, -684.5681)
  line L26 (24.8103, -684.5681) -> (24.8103, -685.1547)
  line L27 (24.8103, -685.1547) -> (22.8151, -685.1548)
  line L28 (22.8151, -685.1548) -> (22.5457, -686.4986)
  spline S86 degree 3 poles (22.5457, -686.4986) (22.6952, -686.4071) (22.986, -686.229) (23.3254, -686.1992) (23.4904, -686.1848) knots 0 0 0 0 0.051785 0.100763 0.100763 0.100763 0.100763
  spline S87 degree 3 poles (23.4904, -686.1848) (23.6997, -686.2031) (24.1153, -686.2396) (24.4361, -686.5061) (24.5955, -686.6384) knots 0 0 0 0 0.061424 0.122014 0.122014 0.122014 0.122014
  spline S88 degree 3 poles (24.5955, -686.6384) (24.7267, -686.8038) (24.9976, -687.1451) (25.0293, -687.5805) (25.0457, -687.8048) knots 0 0 0 0 0.061868 0.127641 0.127641 0.127641 0.127641
  spline S89 degree 3 poles (25.0457, -687.8048) (25.0305, -688.0218) (25.0006, -688.4476) (24.7654, -688.8035) (24.6501, -688.9781) knots 0 0 0 0 0.064036 0.125703 0.125703 0.125703 0.125703
  spline S90 degree 3 poles (24.6501, -688.9781) (24.4723, -689.1551) (24.1093, -689.5168) (23.598, -689.5621) (23.337, -689.5852) knots 0 0 0 0 0.072854 0.148822 0.148822 0.148822 0.148822
  spline S91 degree 3 poles (23.337, -689.5852) (23.1238, -689.5724) (22.7162, -689.5481) (22.3825, -689.3145) (22.2234, -689.2032) knots 0 0 0 0 0.062678 0.119794 0.119794 0.119794 0.119794
  spline S92 degree 3 poles (22.2234, -689.2032) (22.0948, -689.0628) (21.8305, -688.7745) (21.7644, -688.3884) (21.7306, -688.1902) knots 0 0 0 0 0.055877 0.114795 0.114795 0.114795 0.114795
  line L29 (28.1494, -688.1731) -> (28.7531, -688.2516)
  spline S93 degree 3 poles (28.7531, -688.2516) (28.7104, -688.4455) (28.6286, -688.8172) (28.3702, -689.0956) (28.2466, -689.2287) knots 0 0 0 0 0.058356 0.111856 0.111856 0.111856 0.111856
  spline S94 degree 3 poles (28.2466, -689.2287) (28.1005, -689.3317) (27.8004, -689.5431) (27.4337, -689.5686) (27.2456, -689.5817) knots 0 0 0 0 0.052559 0.107965 0.107965 0.107965 0.107965
  spline S95 degree 3 poles (27.2456, -689.5817) (27.0125, -689.5642) (26.5609, -689.5303) (26.2167, -689.2374) (26.0501, -689.0957) knots 0 0 0 0 0.068154 0.132052 0.132052 0.132052 0.132052
  spline S96 degree 3 poles (26.0501, -689.0957) (25.9186, -688.905) (25.6307, -688.4876) (25.6097, -687.9788) (25.5982, -687.7025) knots 0 0 0 0 0.068157 0.149141 0.149141 0.149141 0.149141